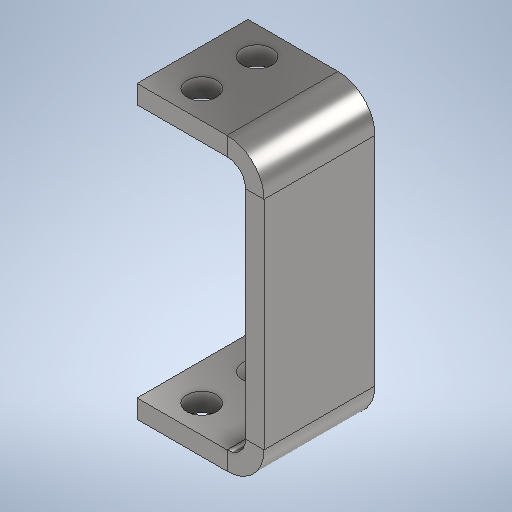
# Autodesk Inventor part: up bracket
Saved by Autodesk Inventor 2026.1 (Build 301233020, 233B)
## iProperties
Created: 2026-01-23
Part Number: up bracket
Material: Steel, Alloy
Document SubType Name: Sheet Metal
Designer: user
Density: 7.73 g/cm^3
Sheet Metal Rule: Default_mm
Appearance: Semi-Polished
Author: user
Autodesk Inventor part; units mm, degrees
ref_plane "YZ Plane" through (0, 0, 0) normal (1, 0, 0) x (0, 1, 0)
ref_plane "XZ Plane" through (0, 0, 0) normal (0, 1, 0) x (-1, 0, 0)
sketch "Sketch1" plane through (0, 0, 0) normal (0, 1, 0) x (-1, 0, 0)
  line L0 (-65, 15) -> (65, 15)
  line L1 (65, 15) -> (65, -15)
  line L2 (65, -15) -> (-65, -15)
  line L3 (-65, -15) -> (-65, 15)
  line L4 (-65, 15) -> (65, -15) construction
  line L5 (65, 15) -> (-65, -15) construction
  point P0 (0, 0)
  dimension "d0" = 130
  dimension "d1" = 30
  measures "d0" distance of L1.end L2.end
  measures "d1" distance of L0.end L1.end
extrude "Plate1" add sketch "Sketch1" along normal blind 5
sketch "Sketch2" plane through (0, 5, 0) normal (0, 1, 0) x (1, 0, 0)
  line L0 (-65, 15) -> (-65, -15) projected
  line L1 (-65, -15) -> (-35, -15)
  line L2 (-65, -15) -> (65, -15) projected
  line L3 (-35, -15) -> (-35, 15)
  line L4 (65, 15) -> (-65, 15) projected
  point P0 (0, 0)
  dimension "d3" = 30
  constraints: 4 end point, 2 point on line, 1 perpendicular
  measures "d3" distance of L0.end L1.end
fold "Fold1" angle 90 bend radius 5 thickness 5 k factor 0.44 line from (-35, 5, 15) to (-35, 5, -15) line at bend centre moving side (1, 0, 0) folds toward (0, 1, 0)
sketch "Sketch3" plane through (0, 5, 0) normal (0, 1, 0) x (1, 0, 0)
  line L0 (-65, -15) -> (-65, 15) projected
  line L1 (-65, 0) -> (-55, 0)
  line L2 (-40.6549, -15) -> (-40.6549, 15) projected
  line L3 (-57.1441, -7.5) -> (-52.8559, -7.5)
  line L4 (-52.8559, -7.5) -> (-52.8559, 7.5)
  line L5 (-52.8559, 7.5) -> (-57.1441, 7.5)
  line L6 (-57.1441, 7.5) -> (-57.1441, -7.5)
  line L7 (-57.1441, -7.5) -> (-52.8559, 7.5) construction
  line L8 (-52.8559, -7.5) -> (-57.1441, 7.5) construction
  circle A0 centre (-55, 7.5) radius 4
  circle A1 centre (-55, -7.5) radius 4
  point P0 (0, 0)
  dimension "d10" = 10
  dimension "d11" = 15
  dimension "d12" = 8
  dimension "d13" = 8
  constraints: 14 end point, 5 midpoint, 2 centre point, 2 parallel, 2 perpendicular, 1 horizontal
  measures "d10" distance of L1.start L1.end
  measures "d11" distance of L4.end L3.end
  measures "d12" diameter of A0
  measures "d13" diameter of A1
extrude "Cut1" cut sketch "Sketch3" against normal blind 5 contours L6 A1 L4 L3 | L3 L4 A1 L6 | A0 L6 L5 L4 | L4 L5 L6 A0
sketch "Sketch7" plane through (-35.6549, 10, 15) normal (-1, 0, 0) x (0, 0, 1)
  line L0 (0, 94.3451) -> (-30, 94.3451) projected
  line L1 (-30, 94.3451) -> (-30, 64.3451)
  line L2 (-30, 94.3451) -> (-30, 0) projected
  line L3 (-30, 64.3451) -> (0, 64.3451)
  line L4 (0, 0) -> (0, 94.3451) projected
  point P0 (-15, -10)
  dimension "d28" = 30
  constraints: 4 end point, 2 point on line, 1 perpendicular
  measures "d28" distance of L0.end L1.end
fold "Fold2" angle 90 bend radius 5 thickness 5 k factor 0.44 line from (-35.6549, 74.3451, -15) to (-35.6549, 74.3451, 15) line at bend centre moving side (0, 1, 0) folds toward (-1, 0, 0)
ref_plane "Work Plane1" through (0, 39.345, 0) normal (0, 1, 0) x (1, 0, 0)
mirror "Mirror1" about plane through (0, 39.345, 0) normal (0, 1, 0) of "Cut1"
sketch "Sketch8" plane through (-65, 73.6903, 15) normal (0, -1, 0) x (1, 0, 0)
  circle A0 centre (10, -7.5) radius 4 projected
  circle A1 centre (10, -7.5) radius 4
  circle A2 centre (10, -22.5) radius 4 projected
  circle A3 centre (10, -22.5) radius 4
  point P0 (65, -15)
  constraints: 2 centre point, 2 coincident
extrude "Cut4" cut sketch "Sketch8" against normal blind 5
equation "\"d2\" = Thickness"
equation "\"d4\" = BendReliefWidth"
equation "\"d5\" = BendReliefDepth"
equation "\"d6\" = MinimumRemnant"
equation "\"d7\" = TransitionRadius"
equation "\"d9\" = BendRadius"
equation "\"d14\" = Thickness"
equation "\"d29\" = BendReliefWidth"
equation "\"d30\" = BendReliefDepth"
equation "\"d31\" = MinimumRemnant"
equation "\"d32\" = TransitionRadius"
equation "\"d34\" = BendRadius"
equation "\"d36\" = Thickness"
equation "\"BendRadius\" = Thickness"
equation "\"BendReliefWidth\" = Thickness"
equation "\"BendReliefDepth\" = 0.5 * Thickness"
equation "\"TransitionRadius\" = BendRadius"
equation "\"JacobiRadiusSize\" = BendRadius"
equation "\"GapSize\" = Thickness"
equation "\"Thickness\" = 5"
equation "\"MinimumRemnant\" = 10"
body "Solid1"
